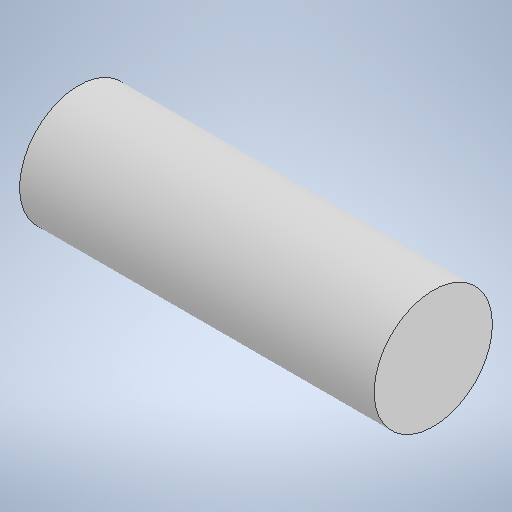
# Autodesk Inventor part: 207 part 3
Saved by Autodesk Inventor 2025.1 (Build 291241000, 241)
## iProperties
Created: 2024-08-23
Part Number: 207 part 3
Material: Generisch
Document SubType Name: Modeling
Designer: ffogue
Density: 1 g/cm^3
Appearance: Vorgabe
Author: ffogue
Autodesk Inventor part; units mm, degrees
ref_plane "YZ Plane" through (0, 0, 0) normal (1, 0, 0) x (0, 1, 0)
ref_plane "XZ Plane" through (0, 0, 0) normal (0, 1, 0) x (-1, 0, 0)
ref_plane "XY Plane" through (0, 0, 0) normal (0, 0, 1) x (1, 0, 0)
sketch "Sketch1" plane through (0, 0, 0) normal (0, 0, 1) x (1, 0, 0)
  line L0 (0, 0) -> (0, 2)
  line L1 (0, 2) -> (12, 2)
  line L2 (12, 2) -> (12, 0)
  line L3 (12, 0) -> (0, 0)
  dimension "d0" = 4
  dimension "d1" = 12
  constraints: 8 end point, 2 perpendicular, 1 parallel, 1 vertical
  measures "d0" diameter of L1 L3
  measures "d1" distance of L0.end L1.end
revolve "Revolution1" add sketch "Sketch1" angle 360 about axis through (12, 0, 0) along (-1, 0, 0)
body "Solid1"
